E_motor_cable_holder_v7 (Autodesk Fusion 360 design; units mm, degrees)
Autodesk Fusion 360 part; units mm, degrees
sketch "Sketch1" plane through (0, 0, 0) normal (0, 0, 1) x (1, 0, 0)
  line L0 (8.5, 17) -> (-8.5, 17)
  line L1 (-8.5, 17) -> (-8.5, -12)
  line L2 (-3.5, -17) -> (3.5, -17)
  line L3 (8.5, -12) -> (8.5, 17)
  line L4 (8.5, 17) -> (-8.5, -17) construction
  line L5 (-8.5, 17) -> (8.5, -17) construction
  line L6 (0, -17) -> (0, 17) construction
  line L7 (-3.5, 17) -> (3.5, 17)
  line L8 (8.5, 12) -> (8.5, 2)
  line L9 (8.5, 2) -> (-8.5, 2)
  line L10 (-8.5, 2) -> (-8.5, 12)
  circle A0 centre (0, -8.5) radius 4.5 construction
  line L11 (-2.0097, -4) -> (2.3533, -4) construction
  line L12 (0, 2) -> (0, 17) construction
  circle A1 centre (0, -8.5) radius 2.7
  line L13 (-8.5, 4) -> (8.5, 4)
  arc A2 (-3.5, 17) -> (-8.5, 12) centre (-3.5, 12) ccw
  arc A3 (8.5, 12) -> (3.5, 17) centre (3.5, 12) ccw
  arc A4 (3.5, -17) -> (8.5, -12) centre (3.5, -12) ccw
  arc A5 (-8.5, -12) -> (-3.5, -17) centre (-3.5, -12) ccw
  point P0 (-8.5, 17)
  point P1 (8.5, 17)
  dimension "d4" = 9
  dimension "d12" = 8.5
  dimension "d13" = 15
  dimension "d14" = 17
  dimension "d15" = 5.4
  dimension "d16" = 10.5
  dimension "d37" = 17
  dimension "d38" = 2
  dimension "d39" = 8.5
  dimension "d43" = 5
  dimension "d44" = 5
  constraint horizontal L0
  constraint perpendicular L0 L1
  constraint parallel L0 L2
  constraint coincident L4 origin
  constraint coincident L5 origin
  constraint midpoint L0 L6.end
  constraint perpendicular L0 L6
  constraint coincident L2 L6.start
  constraint horizontal L7
  constraint vertical L8
  constraint horizontal L9
  constraint vertical L10
  constraint perpendicular L3 L11
  constraint tangent A0 L11
  constraint midpoint L9 L12.start
  constraint collinear L6 L12
  constraint concentric A0 A1
  constraint coincident L6 A0.centre
  constraint vertical L3
  constraint coincident L10 L13.start
  constraint coincident L8 L13.end
  constraint perpendicular L8 L13
  constraint collinear L0 L7
  constraint coincident L7 L6.end
  constraint coincident P0 L7
  constraint coincident P0 L10
  constraint tangent L7 A2
  constraint tangent L10 A2
  constraint coincident P1 L7
  constraint coincident P1 L8
  constraint tangent L7 A3
  constraint tangent L8 A3
  constraint equal A2 A3
  constraint coincident L5.end L2
  constraint coincident L5.end L3
  constraint tangent L2 A4
  constraint tangent L3 A4
  constraint equal A2 A4
  constraint coincident L4.end L1
  constraint coincident L4.end L2
  constraint tangent L1 A5
  constraint tangent L2 A5
  measures "d4" diameter of A0
  measures "d12" distance of L3 A0.centre
  measures "d13" distance of P1 L8.end
  measures "d14" distance of P0 P1
  measures "d15" diameter of A1
  measures "d16" distance of L9 A0.centre
  measures "d37" distance of L4.end L5.end
  measures "d38" distance of L9 L13
  measures "d39" distance of L2 A0.centre
  measures "d43" radius of A2
  measures "d44" radius of A5
extrude "Extrude1" add sketch "Sketch1" along normal blind 2 contours L0 L1 L3 L7 L8 L10 L13 A2 A3 | L1 L3 L8 L9 L10 L13 | L1 L2 L3 L9 A4 A5
extrude "Extrude2" add sketch "Sketch1" along normal blind 6 from surface at 2 contours L1 L3 L8 L9 L10 L13
extrude "Extrude4" add sketch "Sketch1" along normal blind 2 from surface at 8 contours L0 L1 L3 L7 L8 L10 L13 A2 A3 | L1 L3 L8 L9 L10 L13
fillet "Fillet2" radius 3 2 edges at (0, 2, 10) (0, 2, 2)
fillet "Fillet2" radius 1 2 edges at (8.5, 4, 5) (-8.5, 4, 5)
equation "spacing = 4 mm"
equation "d8 = ( d4 / 2 ) + spacing"
equation "d12 = ( d4 / 2 ) + spacing"
equation "d14 = d37"
equation "d39 = d12"
equation "d44 = d43"
